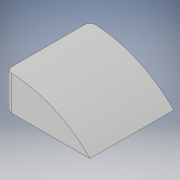
# Autodesk Inventor part: linear_stop_brackets
Saved by Autodesk Inventor 2019.4 (Build 234330000, 330)
## iProperties
Created: 2020-10-31
Part Number: linear_stop_brackets
Material: Generic
Document SubType Name: Modeling
Designer: deanv
Density: 1 g/cm^3
Appearance: Default
Author: deanv
Autodesk Inventor part; units mm, degrees
ref_plane "YZ Plane" through (0, 0, 0) normal (1, 0, 0) x (0, 1, 0)
ref_plane "XZ Plane" through (0, 0, 0) normal (0, 1, 0) x (-1, 0, 0)
ref_plane "XY Plane" through (0, 0, 0) normal (0, 0, 1) x (1, 0, 0)
sketch "Sketch1" plane through (0, 0, 0) normal (0, 0, 1) x (1, 0, 0)
  line L0 (-15, -6.25) -> (15, -6.25)
  line L1 (15, -6.25) -> (15, 6.25)
  line L2 (15, 6.25) -> (-15, 6.25)
  line L3 (-15, 6.25) -> (-15, -6.25)
  line L4 (-15, -6.25) -> (15, 6.25) construction
  line L5 (15, -6.25) -> (-15, 6.25) construction
  arc A0 (15, -6.25) -> (-15, 6.25) centre (-15, -36) ccw
  point P0 (0, 0)
  dimension "d0" = 30
  dimension "d1" = 12.5
  constraints: 12 end point, 2 midpoint, 2 parallel, 2 point on circle, 1 centre point, 1 horizontal, 1 perpendicular, 1 tangent
  measures "d0" distance of L2.end L1.end
  measures "d1" distance of L1.end L0.end
extrude "Extrusion1" add sketch "Sketch1" along normal blind 30 contours L3 A0 L0
fillet "Fillet1" radius 2 2 edges at (-15, 0, 30) (-15, 0, 0)
body "Solid1"
